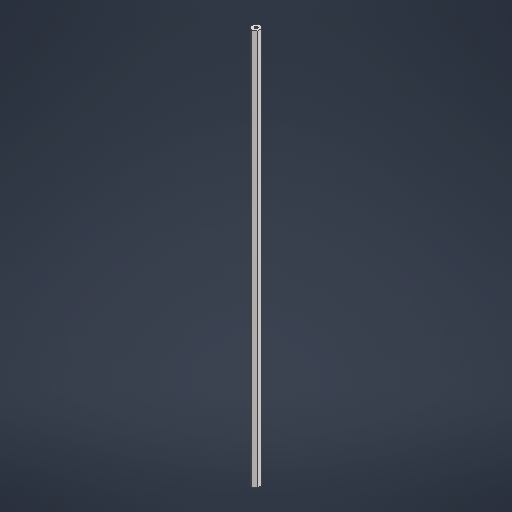
# Autodesk Inventor part: EIXO SEXTAVADO 661,4MM
Saved by Autodesk Inventor 2026 (Build 300175000, 175)
## iProperties
Created: 2026-06-25
Part Number: EIXO SEXTAVADO 661,4MM
Material: Genérico
Document SubType Name: Modeling
Designer: DELL
Density: 1 g/cm^3
Appearance: Padrão
Author: DELL
Autodesk Inventor part; units mm, degrees
ref_plane "YZ Plane" through (0, 0, 0) normal (1, 0, 0) x (0, 1, 0)
ref_plane "XZ Plane" through (0, 0, 0) normal (0, 1, 0) x (-1, 0, 0)
ref_plane "XY Plane" through (0, 0, 0) normal (0, 0, 1) x (1, 0, 0)
sketch "Esboço1" plane through (0, 0, 0) normal (0, 1, 0) x (-1, 0, 0)
  line L0 (0, -7.3323) -> (-6.35, -3.6662)
  line L1 (-6.35, -3.6662) -> (-6.35, 3.6662)
  line L2 (-6.35, 3.6662) -> (0, 7.3323)
  line L3 (0, 7.3323) -> (6.35, 3.6662)
  line L4 (6.35, 3.6662) -> (6.35, -3.6662)
  line L5 (6.35, -3.6662) -> (0, -7.3323)
  point P0 (0, 0)
  point P1 (0, 0)
  dimension "d0" = 12.7
  constraints: 12 end point, 1 coincident, 13 other
  measures "d0" distance between parallel lines of L0 L3
extrude "Extrusão1" add sketch "Esboço1" along normal blind 661.4
sketch "Esboço2" plane through (0, 661.4, 0) normal (0, 1, 0) x (1, 0, 0)
  circle A0 centre (0, 0) radius 2.5
  dimension "d3" = 5
  constraints: 1 centre point, 1 coincident
  measures "d3" diameter of A0
extrude "Extrusão2" cut sketch "Esboço2" against normal blind 1
